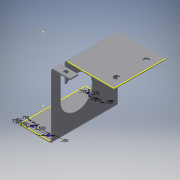
# Autodesk Inventor part: Tape Measure Dispenser Side 1
Saved by Autodesk Inventor 2016 (Build 200138000, 138)
## iProperties
Created: 2016-02-03
Part Number: Tape Measure Dispenser Side 1
Material: Generic
Document SubType Name: Sheet Metal
Designer: GEH-Magnet School 1
Density: 1 g/cm^3
Sheet Metal Rule: Default
Appearance: Default
Author: GEH-Magnet School 1
Autodesk Inventor part; units mm, degrees
note: some values were not read from the file. Chosen so that the rebuilt part matches the saved one: flange form of "Plate2".
ref_plane "YZ Plane" through (0, 0, 0) normal (1, 0, 0) x (0, 1, 0)
ref_plane "XZ Plane" through (0, 0, 0) normal (0, 1, 0) x (-1, 0, 0)
ref_plane "XY Plane" through (0, 0, 0) normal (0, 0, 1) x (1, 0, 0)
sketch "Sketch1" plane through (0, 0, 0) normal (0, 1, 0) x (-1, 0, 0)
  line L0 (-9.2054, 64.0966) -> (-85.4054, 64.0966)
  line L1 (-85.4054, 64.0966) -> (-85.4054, -88.3034)
  line L2 (-85.4054, -88.3034) -> (-9.2054, -88.3034)
  line L3 (-9.2054, -88.3034) -> (-9.2054, 64.0966)
  point P0 (0, 0)
  dimension "d0" = 152.4
  dimension "d1" = 76.2
  measures "d0" distance of L0.end L1.end
  measures "d1" distance of L0.start L0.end
extrude "Plate1" add sketch "Sketch1" along normal blind 3.048
sketch "Sketch2" plane through (82.3574, 0, -88.3034) normal (1, 0, 0) x (0, 1, 0)
  line L0 (0, 152.4) -> (0, 0)
  line L1 (0, 0) -> (152.4, 0)
  line L2 (152.4, 0) -> (152.4, 152.4)
  line L3 (152.4, 152.4) -> (0, 152.4)
  constraints: 6 end point, 1 horizontal, 1 perpendicular, 1 vertical
edge flange "Flange1" height 152.4 angle 90 thickness 3.048 bend radius 3.048 thickness toward (1, 0, 0) relief tear relief width 3.048 relief depth 1.524 edges at (85.4054, 3.048, -12.1034) wall of the first edge with corners at (82.3574, 0, 64.0966) (82.3574, 0, -88.3034) (82.3574, 152.4, -88.3034) (82.3574, 152.4, 64.0966)
bend "Bend1"
corner "Corner1"
sketch "Sketch3" plane through (85.4054, 152.4, 64.0966) normal (1, 0, 0) x (0, 0, -1)
  circle A0 centre (57.15, -76.2) radius 38.1
  line L0 (152.4, 0) -> (152.4, -146.304) projected
  line L1 (152.4, -152.4) -> (0, -152.4) projected
  point P0 (64.0966, -152.4)
  dimension "d13" = 76.2
  dimension "d14" = 95.25
  dimension "d15" = 76.2
  constraints: 1 centre point
  measures "d13" diameter of A0
  measures "d14" distance from line of L0 A0.centre
  measures "d15" distance from line of L1 A0.centre
extrude "Cut1" cut sketch "Sketch3" against normal blind 3.048
sketch "Sketch4" plane through (85.4054, 152.4, 64.0966) normal (1, 0, 0) x (0, 0, -1)
  circle A0 centre (57.15, -76.2) radius 38.1 projected
  line L0 (19.05, -76.2) -> (19.05, 0)
  line L1 (19.05, 0) -> (31.75, 0)
  line L2 (0, 0) -> (152.4, 0) projected
  line L3 (19.05, 0) -> (31.75, 0)
  line L4 (31.75, 0) -> (31.75, -47.8019)
  arc A1 (31.75, -47.8019) -> (19.05, -76.2) centre (57.15, -76.2) ccw
  point P0 (64.0966, -152.4)
  dimension "d18" = 12.7
  constraints: 8 end point, 4 point on circle, 1 centre point, 1 collinear, 1 concentric, 1 perpendicular, 1 point on line, 1 tangent, 1 vertical
  measures "d18" distance of L1.end L0.end
extrude "Cut2" cut sketch "Sketch4" against normal blind 3.048 contours A0 L0 L1 L4
sketch "Sketch5" plane through (82.3574, 149.352, 32.3466) normal (0, 1, 0) x (-1, 0, 0)
  line L0 (0, -120.65) -> (0, 0)
  line L1 (0, 0) -> (-114.3, 0)
  line L2 (-114.3, 0) -> (-114.3, -120.65)
  line L3 (-114.3, -120.65) -> (0, -120.65)
  constraints: 6 end point, 1 horizontal, 1 perpendicular, 1 vertical
edge flange "Flange2" height 114.3 angle 90 thickness 3.048 bend radius 3.048 thickness toward (0, 1, 0) relief tear relief width 3.048 relief depth 1.524 edges at (85.4054, 152.4, -27.9784) wall of the first edge with corners at (82.3574, 149.352, -88.3034) (82.3574, 149.352, 32.3466) (196.6574, 149.352, 32.3466) (196.6574, 149.352, -88.3034)
bend "Bend2"
corner "Corner2"
sketch "Sketch6" plane through (196.6574, 152.4, 32.3466) normal (0, 1, 0) x (1, 0, 0)
  line L0 (0, 120.65) -> (0, 0) projected
  line L1 (0, 0) -> (-108.204, 0) projected
  point P0 (-196.6574, 32.3466)
sketch "Sketch7" plane through (82.3574, 149.352, 64.0966) normal (0, 1, 0) x (-1, 0, 0)
  line L0 (0, -19.05) -> (0, 0)
  line L1 (0, 0) -> (-44.45, 0)
  line L2 (-44.45, 0) -> (-44.45, -19.05)
  line L3 (-44.45, -19.05) -> (0, -19.05)
  constraints: 6 end point, 1 horizontal, 1 perpendicular, 1 vertical
edge flange "Flange3" height 44.45 angle 90 thickness 3.048 bend radius 3.048 thickness toward (0, 1, 0) relief tear relief width 3.048 relief depth 1.524 edges at (85.4054, 152.4, 54.5716) wall of the first edge with corners at (82.3574, 149.352, 45.0466) (82.3574, 149.352, 64.0966) (126.8074, 149.352, 64.0966) (126.8074, 149.352, 45.0466)
bend "Bend3"
corner "Corner3"
sketch "Sketch8" plane through (196.6574, 152.4, 32.3466) normal (0, 1, 0) x (1, 0, 0)
  circle A0 centre (-19.05, 95.25) radius 6.35
  line L0 (0, 120.65) -> (0, 0) projected
  circle A1 centre (-19.05, 25.4) radius 6.35 projected
  point P0 (-196.6574, 32.3466)
  dimension "d46" = 12.7
  dimension "d47" = 19.05
  dimension "d48" = 69.85
  constraints: 1 centre point
  measures "d46" diameter of A0
  measures "d47" distance from line of L0 A0.centre
  measures "d48" distance of A1.centre A0.centre
extrude "Cut4" cut sketch "Sketch8" against normal blind 3.048 contours A0
sketch "Sketch9" plane through (126.8074, 152.4, 64.0966) normal (0, 1, 0) x (1, 0, 0)
  circle A0 centre (-19.05, 9.525) radius 4.7625
  line L0 (0, 0) -> (-38.354, 0) projected
  line L1 (0, 19.05) -> (0, 0) projected
  point P0 (-126.8074, 64.0966)
  dimension "d51" = 9.525
  dimension "d52" = 9.525
  dimension "d53" = 19.05
  constraints: 1 centre point
  measures "d51" diameter of A0
  measures "d52" distance from line of L0 A0.centre
  measures "d53" distance from line of L1 A0.centre
extrude "Cut5" cut sketch "Sketch9" against normal blind 3.048
sketch "Sketch10" plane through (196.6574, 152.4, 32.3466) normal (0, 1, 0) x (1, 0, 0)
  circle A0 centre (-19.05, 25.4) radius 6.35
  line L0 (0, 120.65) -> (0, 0) projected
  circle A1 centre (-19.05, 95.25) radius 6.35 projected
  point P0 (-196.6574, 32.3466)
  dimension "d56" = 12.7
  dimension "d57" = 19.05
  dimension "d58" = 69.85
  constraints: 1 centre point
  measures "d56" diameter of A0
  measures "d57" distance from line of L0 A0.centre
  measures "d58" distance of A1.centre A0.centre
extrude "Cut6" cut sketch "Sketch10" against normal blind 3.048 contours A0
sketch "Sketch11" plane through (0, 3.048, 0) normal (0, 1, 0) x (1, 0, 0)
  circle A0 centre (28.2554, -54.5716) radius 3.175
  circle A1 centre (66.3554, -54.5716) radius 3.175
  line L0 (79.3094, -64.0966) -> (9.2054, -64.0966) projected
  line L1 (9.2054, -64.0966) -> (9.2054, 88.3034) projected
  line L2 (9.2054, 88.3034) -> (79.3094, 88.3034) projected
  circle A2 centre (28.2554, 78.7784) radius 3.175
  circle A3 centre (66.3554, 81.9534) radius 3.175
  point P0 (0, 0)
  dimension "d61" = 6.35
  dimension "d62" = 6.35
  dimension "d63" = 38.1
  dimension "d64" = 9.525
  dimension "d65" = 9.525
  dimension "d67" = 19.05
  dimension "d68" = 9.525
  dimension "d69" = 6.35
  dimension "d70" = 19.05
  dimension "d71" = 6.35
  dimension "d72" = 6.35
  constraints: 4 centre point, 2 coincident
  measures "d61" diameter of A0
  measures "d62" diameter of A1
  measures "d63" distance of A1.centre A0.centre
  measures "d64" distance from line of L0 A1.centre
  measures "d65" distance from line of L0 A0.centre
  measures "d67" distance from line of L1 A0.centre
  measures "d68" distance from line of point (28.255, 78.778) L2
  measures "d69" distance from line of L2 point (66.355, 81.953)
  measures "d70" distance from line of L1 point (28.255, 78.778)
  measures "d71" diameter of A2
  measures "d72" diameter of A3
sketch "Sketch12" plane through (0, 3.048, 0) normal (0, 1, 0) x (1, 0, 0)
  circle A0 centre (66.3554, 78.7784) radius 3.175
  line L0 (9.2054, 88.3034) -> (79.3094, 88.3034) projected
  line L1 (9.2054, -64.0966) -> (9.2054, 88.3034) projected
  point P0 (0, 0)
  dimension "d73" = 6.35
  dimension "d74" = 9.525
  dimension "d75" = 57.15
  constraints: 1 centre point
  measures "d73" diameter of A0
  measures "d74" distance from line of A0.centre L0
  measures "d75" distance from line of A0.centre L1
extrude "Cut7" cut sketch "Sketch11" against normal blind 3.048 contours A0 | A1 | A2
hole "Hole1" at (66.3554, 3.048, -78.7784) direction (0, -1, 0) diameter 6.35 depth 3.048 tip angle 118
equation "\"d16\" = Thickness"
equation "\"d19\" = Thickness"
equation "\"d49\" = Thickness"
equation "\"d54\" = Thickness"
equation "\"d59\" = Thickness"
equation "\"d76\" = Thickness"
equation "\"d83\" = Thickness"
equation "\"d3\" = BendReliefWidth"
equation "\"d4\" = BendReliefDepth"
equation "\"d5\" = MinimumRemnant"
equation "\"d6\" = BendRadius"
equation "\"d9\" = BendRadius"
equation "\"d10\" = CornerReliefSize"
equation "\"d11\" = GapSize"
equation "\"d12\" = JacobiRadiusSize"
equation "\"d21\" = BendReliefWidth"
equation "\"d22\" = BendReliefDepth"
equation "\"d23\" = MinimumRemnant"
equation "\"d24\" = BendRadius"
equation "\"d27\" = BendRadius"
equation "\"d28\" = CornerReliefSize"
equation "\"d29\" = GapSize"
equation "\"d30\" = JacobiRadiusSize"
equation "\"d34\" = BendReliefWidth"
equation "\"d35\" = BendReliefDepth"
equation "\"d36\" = MinimumRemnant"
equation "\"d37\" = BendRadius"
equation "\"d40\" = BendRadius"
equation "\"d41\" = CornerReliefSize"
equation "\"d42\" = GapSize"
equation "\"d43\" = JacobiRadiusSize"
equation "\"BendRadius\" = Thickness"
equation "\"BendReliefWidth\" = Thickness"
equation "\"BendReliefDepth\" = 0.5 * Thickness"
equation "\"CornerReliefSize\" = 4 * Thickness"
equation "\"MinimumRemnant\" = 2 * Thickness"
equation "\"TransitionRadius\" = BendRadius"
equation "\"JacobiRadiusSize\" = BendRadius"
equation "\"GapSize\" = Thickness"
equation "\"d2\" = BendRadius"
equation "\"Thickness\" = 3.048"
body "Solid1"
